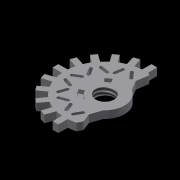
# Autodesk Inventor part: ShoulderCogSmall
Saved by Autodesk Inventor 2015 (Build 190159000, 159)
## iProperties
RuleStatus: InUse
Created: 2014-09-25
Part Number: ShoulderCogSmall
Material: Generic
Document SubType Name: Modeling
Designer: Inventor
Mass: 0.498803 g
Surface Area: 9.11002 cm^2
Volume: 0.498803 cm^3
Density: 1 g/cm^3
Appearance: Default
BeforeDocSave0: UpdateBoundingBox
CX: 18.48 mm
CY: 26.46 mm
CZ: 2.00 mm
Author: Inventor
Autodesk Inventor part; units mm, degrees
ref_plane "YZ Plane" through (0, 0, 0) normal (1, 0, 0) x (0, 1, 0)
ref_plane "XZ Plane" through (0, 0, 0) normal (0, 1, 0) x (-1, 0, 0)
ref_plane "XY Plane" through (0, 0, 0) normal (0, 0, 1) x (1, 0, 0)
sketch "Body" plane through (0, 0, 0) normal (0, 0, 1) x (1, 0, 0)
  circle A0 centre (0, 0) radius 13.25 construction
  circle A1 centre (0, 0) radius 10.75
  line L0 (0, 0) -> (0, 13.25) construction
  line L1 (-0.75, 13.2288) -> (0.75, 13.2288)
  line L2 (-0.75, 13.2288) -> (-0.7938, 10.7207)
  line L3 (0.75, 13.2288) -> (0.7938, 10.7207)
  line L4 (-0.7938, 10.7207) -> (0.7938, 10.7207)
  point P0 (0, 13.2288)
  dimension "d0" = 26.5
  dimension "d1" = 2.5
  dimension "d2" = 1.5
  dimension "d3" = 91
  dimension "d4" = 91
  constraints: 10 end point, 4 point on circle, 2 centre point, 2 coincident, 1 horizontal, 1 midpoint, 1 point on line, 1 vertical
  measures "d0" diameter of A0
  measures "d1" radial gap between concentric circles of A0 A1
  measures "d2" distance of L1.start L1.end
  measures "d3" angle of L1 L2
  measures "d4" angle of L1 L3
extrude "BodyFeature" add sketch "Body" along normal blind 2 contours A1 L4 picked at (2.6338, -2.2653)
sketch "Tooth" plane through (0, 0, 0) normal (0, 0, -1) x (-1, 0, 0)
  line L0 (0.75, 13.2288) -> (0.7938, 10.7207) projected
  line L1 (0.75, 13.2288) -> (-0.75, 13.2288) projected
  line L2 (-0.75, 13.2288) -> (-0.7938, 10.7207) projected
  line L3 (0.7938, 10.7207) -> (-0.7938, 10.7207) projected
extrude "ToothFeature" add sketch "Tooth" against normal blind 2
pattern_circular "ToothArray" count 11 over 180 about axis through (0, 0, 0) along (0, 0, 1) of "ToothFeature"
sketch "Sketch3" plane through (0, 0, 0) normal (0, 0, -1) x (-1, 0, 0)
  point P0 (0, 0)
hole "BodyHole" at (0, 0, 0) direction (0, 0, 1) diameter 4.917 end through all thread size "M6x1" class "6H" standard "ISO Metric profile"
sketch "BodyCutDetail" plane through (0, 0, 2) normal (0, 0, 1) x (1, 0, 0)
  circle A0 centre (0, 0) radius 2.4585 construction
  line L0 (-6.7837, 5.7279) -> (-3.8206, 5.2586) construction
  line L1 (-3.8206, 5.2586) -> (-3.3513, 8.2217) construction
  line L2 (-3.8206, 5.2586) -> (0, 0) construction
  circle A1 centre (-3.3513, 8.2217) radius 0.4
  circle A2 centre (-6.7837, 5.7279) radius 0.4
  circle A3 centre (-3.6642, 6.2463) radius 0.4
  circle A4 centre (-4.8083, 5.415) radius 0.4
  line L3 (-3.3513, 8.2217) -> (-3.6642, 6.2463) construction
  line L4 (-4.8083, 5.415) -> (-6.7837, 5.7279) construction
  line L5 (-2.9562, 8.1591) -> (-3.2691, 6.1837)
  line L6 (-3.7464, 8.2842) -> (-4.0592, 6.3089)
  line L7 (-4.7457, 5.8101) -> (-6.7211, 6.123)
  line L8 (-4.8709, 5.02) -> (-6.8462, 5.3328)
  line L9 (-3.8206, 5.2586) -> (-7.7757, 10.7023) construction
  line L10 (-7.1689, 11.1431) -> (-8.3824, 10.2614) construction
  circle A5 centre (-7.852, 4.144) radius 0.4
  circle A6 centre (-8.8784, 0.0274) radius 0.4
  circle A7 centre (-6.822, 2.4297) radius 0.4
  circle A8 centre (-7.1641, 1.0575) radius 0.4
  line L11 (-7.5092, 4.35) -> (-6.4791, 2.6357)
  line L12 (-8.1949, 3.938) -> (-7.1648, 2.2236)
  line L13 (-7.3701, 1.4003) -> (-9.0844, 0.3702)
  line L14 (-6.9581, 0.7146) -> (-8.6724, -0.3155)
  circle A9 centre (-8.6787, -1.8727) radius 0.4
  circle A10 centre (-6.8189, -5.686) radius 0.4
  circle A11 centre (-6.7877, -2.5238) radius 0.4
  circle A12 centre (-6.1677, -3.7949) radius 0.4
  line L15 (-8.5485, -1.4945) -> (-6.6575, -2.1456)
  line L16 (-8.8089, -2.2509) -> (-6.9179, -2.9021)
  line L17 (-6.5459, -3.6647) -> (-7.1971, -5.5557)
  line L18 (-5.7895, -3.9252) -> (-6.4407, -5.8162)
  circle A13 centre (-5.4445, -7.0131) radius 0.4
  circle A14 centre (-1.5687, -8.7388) radius 0.4
  circle A15 centre (-3.5774, -6.2964) radius 0.4
  circle A16 centre (-2.2854, -6.8716) radius 0.4
  line L19 (-5.5879, -6.6397) -> (-3.7207, -5.923)
  line L20 (-5.3012, -7.3866) -> (-3.434, -6.6698)
  line L21 (-2.6589, -7.015) -> (-1.9421, -8.8821)
  line L22 (-1.912, -6.7283) -> (-1.1953, -8.5954)
  circle A17 centre (0.3372, -8.8721) radius 0.4
  circle A18 centre (4.4155, -7.7026) radius 0.4
  circle A19 centre (1.3068, -7.1228) radius 0.4
  circle A20 centre (2.6663, -6.733) radius 0.4
  line L23 (-0.0126, -8.6781) -> (0.957, -6.9289)
  line L24 (0.6871, -9.066) -> (1.6567, -7.3167)
  line L25 (2.4723, -7.0829) -> (4.2216, -8.0525)
  line L26 (2.8602, -6.3832) -> (4.6094, -7.3528)
  circle A21 centre (5.9612, -6.5796) radius 0.4
  circle A22 centre (8.3336, -3.0623) radius 0.4
  circle A23 centre (5.5796, -4.6164) radius 0.4
  circle A24 centre (6.3704, -3.4439) radius 0.4
  line L27 (5.5685, -6.656) -> (5.1869, -4.6927)
  line L28 (6.3538, -6.5033) -> (5.9722, -4.5401)
  line L29 (6.4467, -3.8366) -> (8.4099, -3.455)
  line L30 (6.294, -3.0513) -> (8.2573, -2.6697)
  circle A25 centre (8.7958, -1.2085) radius 0.4
  circle A26 centre (8.3524, 3.0109) radius 0.4
  circle A27 centre (7.2415, 0.0501) radius 0.4
  circle A28 centre (7.0937, 1.4566) radius 0.4
  line L31 (8.5441, -1.5194) -> (6.9898, -0.2607)
  line L32 (9.0476, -0.8977) -> (7.4933, 0.361)
  line L33 (7.4046, 1.2049) -> (8.6632, 2.7591)
  line L34 (6.7829, 1.7083) -> (8.0415, 3.2626)
  circle A29 centre (7.5148, 4.7281) radius 0.4
  circle A30 centre (4.4629, 7.6753) radius 0.4
  circle A31 centre (5.5151, 4.6932) radius 0.4
  circle A32 centre (4.4978, 5.6756) radius 0.4
  line L35 (7.5218, 4.3281) -> (5.5221, 4.2932)
  line L36 (7.5078, 5.128) -> (5.5081, 5.0931)
  line L37 (4.8978, 5.6825) -> (4.8629, 7.6822)
  line L38 (4.0979, 5.6686) -> (4.063, 7.6683)
  circle A33 centre (2.7175, 8.4523) radius 0.4
  circle A34 centre (-1.5148, 8.7483) radius 0.4
  circle A35 centre (1.2081, 7.1402) radius 0.4
  circle A36 centre (-0.2026, 7.2389) radius 0.4
  line L39 (2.98, 8.1505) -> (1.4706, 6.8383)
  line L40 (2.4551, 8.7542) -> (0.9457, 7.4421)
  line L41 (0.0992, 7.5013) -> (-1.2129, 9.0107)
  line L42 (-0.5045, 6.9765) -> (-1.8166, 8.4859)
  dimension "d97" = 135
  dimension "d99" = 3
  dimension "d100" = 6.5
  dimension "d101" = 0.8
  dimension "d103" = 135
  dimension "d104" = 1
  dimension "d108" = 360
  constraints: 84 end point, 72 point on circle, 36 centre point, 8 tangent, 3 equal radius, 3 perpendicular, 2 coincident, 2 collinear, 1 midpoint, 181 other
  measures "d97" angle of L1 L2
  measures "d99" distance of L0.start L0.end
  measures "d100" distance of L0.end L2.end
  measures "d101" diameter of A1
  measures "d103" angle of L2 L0
  measures "d104" distance of L0.end L3.end
extrude "BodyCutDetailFeature" cut sketch "BodyCutDetail" against normal through all contours A1 | A1 L5 A3 L6 | A3 | A2 | A2 L7 A4 L8 | A4 | A5 | A5 L11 A7 L12 | A7 | A6 | A6 L13 A8 L14 | A8 | A9 | A9 L15 A11 L16 | A11 | A10 | A10 L17 A12 L18 | A12 | A13 | A13 L19 A15 L20 | A15 | A14 | A14 L21 A16 L22 | A16 | A17 | A17 L23 A19 L24 | A19 | A34 | A34 L41 A36 L42 | A36
sketch "BodyLimitCut" plane through (0, 0, 2) normal (0, 0, 1) x (1, 0, 0)
  circle A0 centre (0, 0) radius 2.4585 construction
  line L0 (0, 0) -> (3.7504, -10.0746) construction
  line L1 (0, 0) -> (1.5738, 10.6342) construction
  arc A1 (0.7938, -10.7207) -> (0.7938, 10.7207) centre (0, 0) ccw construction
  circle A2 centre (0, 0) radius 5.25 construction
  arc A3 (3.7504, -10.0746) -> (1.5738, 10.6342) centre (0, 0) ccw
  arc A4 (1.8316, -4.9201) -> (0.7686, 5.1934) centre (0, 0) ccw
  line L2 (1.8316, -4.9201) -> (3.7504, -10.0746)
  line L3 (0.7686, 5.1934) -> (1.5738, 10.6342)
  point P0 (1.6567, -7.3167)
  point P1 (0.0992, 7.5013)
  dimension "d117" = 1
  dimension "d118" = 1
  dimension "d119" = 10.5
  constraints: 8 end point, 8 point on circle, 3 centre point, 2 concentric, 2 point on line, 1 coincident
  measures "d117" distance from line of L0 point (1.657, -7.317)
  measures "d118" distance from line of L1 point (0.099, 7.501)
  measures "d119" diameter of A2
extrude "BodyLimitCutFeature" cut sketch "BodyLimitCut" against normal through all
chamfer "BodyChamfer1Feature" distance 2 angle 45 1 edges at (0.7686, 5.1934, 1)
chamfer "BodyChamfer2Feature" distance 2 angle 45 1 edges at (1.8316, -4.9201, 1)
chamfer "BodyChamfer3Feature" distance 1 angle 45 1 edges at (3.7504, -10.0746, 1)
chamfer "BodyChamfer4Feature" distance 0.4 angle 45 1 edges at (1.5738, 10.6342, 1)
sketch "BodyDetail" plane through (0, 0, 2) normal (0, 0, 1) x (1, 0, 0)
  circle A0 centre (0, 0) radius 4 construction
  circle A1 centre (0, 0) radius 5.25 construction
  circle A2 centre (0, 0) radius 2.4585 construction
  line L0 (-2.1764, -4.7776) -> (0, 0) construction
  line L1 (0, 0) -> (-4.7021, -2.335) construction
  line L2 (3.5387, -3.8782) -> (2.5293, -6.7945) construction
  arc A3 (-4.7021, -2.335) -> (-2.1764, -4.7776) centre (0, 0) ccw
  arc A4 (-3.5826, -1.7791) -> (-1.6582, -3.6401) centre (0, 0) ccw
  line L3 (-4.7021, -2.335) -> (-3.5826, -1.7791)
  line L4 (-2.1764, -4.7776) -> (-1.6582, -3.6401)
  line L5 (0, 0) -> (-3.8024, 3.6199) construction
  line L6 (0, 0) -> (-2.4977, 4.6178) construction
  arc A5 (-2.4977, 4.6178) -> (-3.8024, 3.6199) centre (0, 0) ccw
  arc A6 (-1.903, 3.5183) -> (-2.8971, 2.758) centre (0, 0) ccw
  line L7 (-3.8024, 3.6199) -> (-2.8971, 2.758)
  line L8 (-1.903, 3.5183) -> (-2.4977, 4.6178)
  dimension "d140" = 8
  dimension "d142" = 5.4
  dimension "d143" = 39.1
  dimension "d144" = 18
  dimension "d145" = 70
  constraints: 17 point on circle, 16 end point, 6 centre point, 5 concentric, 4 point on line, 2 collinear, 1 coincident
  measures "d140" diameter of A0
  measures "d142" angle of L0 L2
  measures "d143" angle of L1 L0
  measures "d144" angle of L6 L5
  measures "d145" angle of L5 L1
extrude "BodyDetailFeature" cut sketch "BodyDetail" against normal blind 1
equation "\"d4\" = d3"
equation "\"d103\" = d97"
